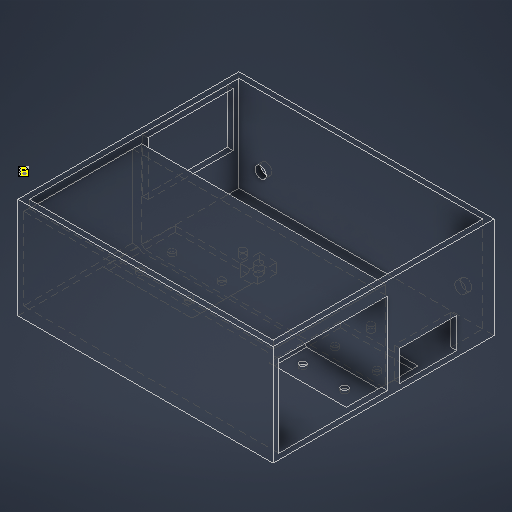
# Autodesk Inventor part: BOTTOM
Saved by Autodesk Inventor 2026.1 (Build 301233020, 233B)
## iProperties
Created: 2026-07-07
Part Number: BOTTOM
Material: Generic
Document SubType Name: Modeling
Designer: pleased
Density: 1 g/cm^3
Appearance: Default
Author: pleased
Autodesk Inventor part; units mm, degrees
ref_plane "YZ Plane" through (0, 0, 0) normal (1, 0, 0) x (0, 1, 0)
ref_plane "XZ Plane" through (0, 0, 0) normal (0, 1, 0) x (-1, 0, 0)
ref_plane "XY Plane" through (0, 0, 0) normal (0, 0, 1) x (1, 0, 0)
sketch "Sketch1" plane through (0, 0, 0) normal (0, 1, 0) x (-1, 0, 0)
  line L0 (0, 120) -> (138, 120)
  line L1 (138, 120) -> (138, 0)
  line L2 (138, 0) -> (0, 0)
  line L3 (0, 0) -> (0, 120)
  point P0 (0, 0)
  dimension "d0" = 138
  dimension "d1" = 120
  constraints: 8 end point, 2 parallel, 1 horizontal, 1 perpendicular
  measures "d0" distance of L1.end L2.end
  measures "d1" distance of L0.end L1.end
extrude "Extrusion1" add sketch "Sketch1" along normal blind 3
sketch "Sketch2" plane through (0, 3, 0) normal (0, 1, 0) x (1, 0, 0)
  circle A0 centre (-123.5, -66.5) radius 1.75
  circle A1 centre (-123.5, -49.5) radius 1.75
  circle A2 centre (-97.5, -66.5) radius 1.75
  circle A3 centre (-97.5, -49.5) radius 1.75
  circle A4 centre (-38, -66.5) radius 1.75
  circle A5 centre (-38, -49.5) radius 1.75
  circle A6 centre (-16, -66.5) radius 1.75
  circle A7 centre (-16, -49.5) radius 1.75
  point P0 (0, 0)
  dimension "d5" = 3.5
  dimension "d6" = 3.5
  dimension "d7" = 3.5
  dimension "d8" = 3.5
  dimension "d9" = 3.5
  dimension "d10" = 3.5
  dimension "d11" = 3.5
  dimension "d12" = 3.5
  constraints: 8 centre point, 8 coincident
  measures "d5" diameter of A0
  measures "d6" diameter of A1
  measures "d7" diameter of A2
  measures "d8" diameter of A3
  measures "d9" diameter of A4
  measures "d10" diameter of A5
  measures "d11" diameter of A6
  measures "d12" diameter of A7
extrude "Extrusion2" cut sketch "Sketch2" against normal blind 3
sketch "Sketch3" plane through (0, 3, 0) normal (0, 1, 0) x (1, 0, 0)
  line L0 (-131.1985, -74.9193) -> (-87.7046, -74.9193)
  line L1 (-87.7046, -74.9193) -> (-87.7046, -40.2677)
  line L2 (-87.7046, -40.2677) -> (-131.1985, -40.2677)
  line L3 (-131.1985, -40.2677) -> (-131.1985, -74.9193)
  line L4 (-44.4498, -74.9193) -> (-6.6914, -74.9193)
  line L5 (-6.6914, -74.9193) -> (-6.6914, -40.2677)
  line L6 (-6.6914, -40.2677) -> (-44.4498, -40.2677)
  line L7 (-44.4498, -40.2677) -> (-44.4498, -74.9193)
  point P0 (0, 0)
  constraints: 16 end point, 4 parallel, 2 horizontal, 2 perpendicular, 2 point on line
extrude "Extrusion3" cut sketch "Sketch3" against normal blind 1.5
chamfer "Chamfer1" distance 1.5 angle 45 8 edges at (-131.1985, 3, 57.5935) (-109.4515, 3, 40.2677) (-109.4515, 3, 74.9193) (-87.7046, 3, 57.5935) (-44.4498, 3, 57.5935) (-25.5706, 3, 40.2677) (-6.6914, 3, 57.5935) (-25.5706, 3, 74.9193)
sketch "Sketch4" plane through (0, 3, 0) normal (0, 1, 0) x (1, 0, 0)
  line L0 (0, 0) -> (-138, 0) projected
  line L1 (-138, -120) -> (0, -120)
  line L2 (0, -120) -> (0, 0)
  line L3 (0, 0) -> (-138, 0)
  line L4 (-138, 0) -> (-138, -120)
  line L5 (-133, -115) -> (-5, -115)
  line L6 (-5, -115) -> (-5, -5)
  line L7 (-5, -5) -> (-133, -5)
  line L8 (-133, -5) -> (-133, -115)
  line L9 (-136, -118) -> (-2, -118)
  line L10 (-2, -118) -> (-2, -2)
  line L11 (-2, -2) -> (-136, -2)
  line L12 (-136, -2) -> (-136, -118)
  dimension "d20" = 5
  dimension "d21" = 3
  constraints: 24 end point, 6 parallel, 3 perpendicular, 1 horizontal, 6 other
  measures "d20" distance between parallel lines of L4 L8
  measures "d21" distance between parallel lines of L8 L12
extrude "Extrusion4" add sketch "Sketch4" along normal blind 50 contours L12 L11 L10 L9
move faces "Move1" translate (0, 0, -2) faces at (-92, 1, 120)
move faces "Move2" translate (-2, 0, 0) faces at (0, 1, 78.6667)
move faces "Move3" translate (0, 0, 2) faces at (-47.3333, 1, 0)
move faces "Move4" translate (2, 0, 0) faces at (-138, 1, 40.6667)
sketch "Sketch7" plane through (0, 3, 0) normal (0, 1, 0) x (1, 0, 0)
  line L0 (-5, -115) -> (-5, -5) projected
  line L1 (-5, -5) -> (-44.335, -5)
  line L2 (-44.335, -5) -> (-44.335, -26.7557)
  line L3 (-44.335, -26.7557) -> (-5, -26.7557)
  line L4 (-5, -26.7557) -> (-5, -5)
  line L5 (-44.335, -26.7557) -> (-84.335, -26.7557)
  line L6 (-84.335, -26.7557) -> (-84.335, -50.7557)
  line L7 (-84.335, -50.7557) -> (-44.335, -50.7557)
  line L8 (-44.335, -50.7557) -> (-44.335, -26.7557)
  line L9 (-84.335, -38.7557) -> (-93.335, -38.7557)
  line L10 (-93.335, -38.7557) -> (-93.335, -33.7557)
  line L11 (-93.335, -33.7557) -> (-84.335, -33.7557)
  line L12 (-84.335, -33.7557) -> (-84.335, -38.7557)
  line L13 (-93.335, -38.7557) -> (-84.335, -38.7557)
  line L14 (-84.335, -38.7557) -> (-84.335, -43.7557)
  line L15 (-84.335, -43.7557) -> (-93.335, -43.7557)
  line L16 (-93.335, -43.7557) -> (-93.335, -38.7557)
  circle A0 centre (-88.835, -38.7557) radius 2
  point P0 (0, 0)
  point P1 (-90.835, -38.7557)
  point P2 (-86.835, -38.7557)
  dimension "d77" = 39.335
  dimension "d78" = 21.7557
  dimension "d79" = 40
  dimension "d80" = 24
  dimension "d81" = 9
  dimension "d82" = 5
  dimension "d83" = 5
  dimension "d84" = 4
  constraints: 32 end point, 8 parallel, 4 horizontal, 4 perpendicular, 2 midpoint, 1 centre point, 1 point on line
  measures "d77" distance of L3.end L2.end
  measures "d78" distance of L2.end L1.end
  measures "d79" distance of L7.end L6.end
  measures "d80" distance of L6.end L5.end
  measures "d81" distance of L10.end L11.end
  measures "d82" distance of L9.end L10.end
  measures "d83" distance of L13.end L14.end
  measures "d84" diameter of A0
extrude "Extrusion7" add sketch "Sketch7" along normal blind 5 and the other way blind 3 contours L6 L9 A0 L10 L11 | L6 L15 L16 L9 A0 | A0 L9 picked at (-88.2253, -39.2251)
sketch "Sketch8" plane through (0, 8, 0) normal (0, 1, 0) x (1, 0, 0)
  line L0 (-90.835, -38.7557) -> (-86.835, -38.7557) projected
  circle A0 centre (-88.835, -38.7557) radius 2
  point P0 (0, 0)
  constraints: 1 midpoint, 3 other
extrude "Extrusion8" cut sketch "Sketch8" against normal blind 5 contours L0 A0 picked at (-88.2253, -39.2251)
sketch "Sketch11" plane through (-5, 3, 5) normal (-1, 0, 0) x (0, 0, 1)
  line L0 (110, 43) -> (70, 43)
  line L1 (70, 43) -> (70, 48)
  line L2 (70, 48) -> (110, 48)
  line L3 (110, 48) -> (110, 43)
  point P0 (-5, -3)
  dimension "d98" = 40
  dimension "d99" = 5
  constraints: 8 end point, 2 parallel, 1 horizontal, 1 perpendicular
  measures "d98" distance of L1.end L2.end
  measures "d99" distance of L0.end L1.end
extrude "Extrusion11" add sketch "Sketch11" along normal blind 130
sketch "Sketch12" plane through (-133, 53, 5) normal (0, 0, 1) x (1, 0, 0)
  line L0 (3.3934, -24.985) -> (123.3934, -24.985)
  line L1 (123.3934, -24.985) -> (123.3934, -48.985)
  line L2 (123.3934, -48.985) -> (3.3934, -48.985)
  line L3 (3.3934, -48.985) -> (3.3934, -24.985)
  line L4 (3.3934, -24.985) -> (11.3934, -24.985)
  line L5 (3.3934, -36.9853) -> (3.3934, -24.985)
  line L6 (3.3934, -24.985) -> (116.3934, -24.985)
  line L7 (3.3934, -36.9853) -> (3.3934, -24.985)
  line L8 (7.3934, -32.9853) -> (15.3934, -32.9853)
  line L9 (15.3934, -32.9853) -> (15.3934, -40.9853)
  line L10 (15.3934, -40.9853) -> (7.3934, -40.9853)
  line L11 (7.3934, -40.9853) -> (7.3934, -32.9853)
  line L12 (15.3934, -32.9853) -> (7.3934, -40.9853) construction
  line L13 (112.3934, -32.9853) -> (120.3934, -32.9853)
  line L14 (120.3934, -32.9853) -> (120.3934, -40.9853)
  line L15 (120.3934, -40.9853) -> (112.3934, -40.9853)
  line L16 (112.3934, -40.9853) -> (112.3934, -32.9853)
  line L17 (112.3934, -32.9853) -> (120.3934, -40.9853) construction
  line L18 (120.3934, -32.9853) -> (112.3934, -40.9853) construction
  circle A0 centre (11.3934, -36.9853) radius 3
  circle A1 centre (116.3934, -36.9853) radius 3
  line L19 (128, -50) -> (0, -50) projected
  point P0 (133, -53)
  dimension "d114" = 120
  dimension "d115" = 24
  dimension "d120" = 8
  dimension "d121" = 8
  dimension "d122" = 8
  dimension "d123" = 8
  dimension "d124" = 6
  dimension "d125" = 6
  dimension "d145" = 1.015
  constraints: 38 end point, 6 parallel, 5 horizontal, 3 perpendicular, 2 centre point, 2 midpoint
  measures "d114" distance of L1.end L2.end
  measures "d115" distance of L0.end L1.end
  measures "d120" distance of L9.end L10.end
  measures "d121" distance of L8.end L9.end
  measures "d122" distance of L14.end L15.end
  measures "d123" distance of L13.end L14.end
  measures "d124" diameter of A0
  measures "d125" diameter of A1
  measures "d145" distance between parallel lines of L19 L2
extrude "Extrusion12" cut sketch "Sketch12" against normal blind 130 contours A0 | A1
sketch "Sketch14" plane through (-136, 0, 2) normal (-1, 0, 0) x (0, 0, 1)
  line L0 (6, 49.8185) -> (50.7, 49.8185)
  line L1 (50.7, 49.8185) -> (50.7, 21.6185)
  line L2 (50.7, 21.6185) -> (6, 21.6185)
  line L3 (6, 21.6185) -> (6, 49.8185)
  line L4 (3, 3) -> (3, 53) projected
  point P0 (-2, 0)
  dimension "d128" = 44.7
  dimension "d129" = 28.2
  dimension "d144" = 3
  constraints: 8 end point, 2 parallel, 1 horizontal, 1 perpendicular
  measures "d128" distance of L1.end L2.end
  measures "d129" distance of L0.end L1.end
  measures "d144" distance between parallel lines of L4 L3
extrude "Extrusion13" cut sketch "Sketch14" against normal blind 25
sketch "Sketch15" plane through (-136, 3, 115) normal (0, 1, 0) x (1, 0, 0)
  circle A0 centre (98, 65.5) radius 1.75 projected
  line L0 (98, 65.5) -> (98, 83)
  line L1 (98, 65.5) -> (115.5, 65.5) construction
  line L2 (98, 83) -> (30.5, 83)
  line L3 (98, 83) -> (99.5, 83)
  line L4 (99.5, 83) -> (32, 83)
  circle A1 centre (32, 83) radius 1.75
  circle A2 centre (99.5, 83) radius 1.75
  point P0 (136, 115)
  dimension "d132" = 17.5
  dimension "d133" = 90
  dimension "d134" = 67.5
  dimension "d135" = 90
  dimension "d136" = 1.5
  dimension "d137" = 67.5
  dimension "d138" = 0
  dimension "d139" = 3.5
  dimension "d140" = 3.5
  constraints: 10 end point, 3 coincident, 2 centre point, 2 horizontal, 2 perpendicular, 1 collinear, 1 vertical
  measures "d132" distance of L0.start L0.end
  measures "d133" angle of L1 L0
  measures "d134" distance of L0.end L2.end
  measures "d135" angle of L2 L0
  measures "d136" distance of L0.end L3.end
  measures "d137" distance of L3.end L4.end
  measures "d138" distance between parallel lines of L4 L3
  measures "d139" diameter of A1
  measures "d140" diameter of A2
extrude "Extrusion14" cut sketch "Sketch15" against normal blind 10 contours A2 L2 L0 | L0 L2 A2 | A1
sketch "Sketch17" plane through (-136, 0, 2) normal (-1, 0, 0) x (0, 0, 1)
  line L0 (113, 3) -> (113, 46) projected
  line L1 (74.4193, 3) -> (36.7677, 3) projected
  line L2 (113, 46) -> (56, 46)
  line L3 (56, 46) -> (56, 3)
  line L4 (56, 3) -> (113, 3)
  line L5 (113, 3) -> (113, 46)
  point P0 (-2, 0)
  dimension "d143" = 57
  constraints: 8 end point, 2 parallel, 1 horizontal, 1 perpendicular, 1 point on line
  measures "d143" distance of L4.end L3.end
extrude "Extrusion15" cut sketch "Sketch17" against normal blind 160
sketch "Sketch18" plane through (-136, 0, 2) normal (-1, 0, 0) x (0, 0, 1)
  line L0 (73, 46) -> (56, 46) projected
  line L1 (56, 46) -> (63, 46)
  line L2 (63, 46) -> (63, 48)
  line L3 (63, 46) -> (65, 46) construction
  line L4 (63, 48) -> (54, 48)
  line L5 (54, 48) -> (54, 42)
  line L6 (54, 42) -> (56, 42)
  line L7 (56, 46) -> (56, 3) projected
  line L8 (56, 42) -> (56, 46)
  point P0 (-2, 0)
  dimension "d148" = 7
  dimension "d150" = 2
  dimension "d151" = 90
  dimension "d152" = 9
  dimension "d153" = 6
  constraints: 14 end point, 6 perpendicular, 2 point on line, 1 horizontal
  measures "d148" distance of L0.end L1.end
  measures "d150" distance of L1.end L2.end
  measures "d151" angle of L3 L2
  measures "d152" distance of L2.end L4.end
  measures "d153" distance of L4.end L5.end
extrude "Extrusion16" add sketch "Sketch18" against normal blind 134
sketch "Sketch19" plane through (-2, 0, 118) normal (1, 0, 0) x (0, 0, -1)
  line L0 (79.2323, 3) -> (41.5807, 3) projected
  line L1 (66.5996, 3) -> (96.3751, 3)
  line L2 (96.3751, 3) -> (96.3751, 18.9395)
  line L3 (96.3751, 18.9395) -> (66.5996, 18.9395)
  line L4 (66.5996, 18.9395) -> (66.5996, 3)
  point P0 (118, 0)
  point P1 (79.2323, 3)
  constraints: 8 end point, 2 parallel, 1 horizontal, 1 perpendicular, 1 point on line
extrude "Extrusion17" cut sketch "Sketch19" against normal blind 25.5
move faces "Move12" translate (0, -41.75, 0) faces at (-47.6667, 42, 56.6667)
move faces "Move13" translate (0, 0, -19) faces at (-47.6667, 49.3333, 75)
move faces "Move14" translate (0, -2.25, 0) faces at (-47.6667, 51, 75.6667)
body "Solid1"
